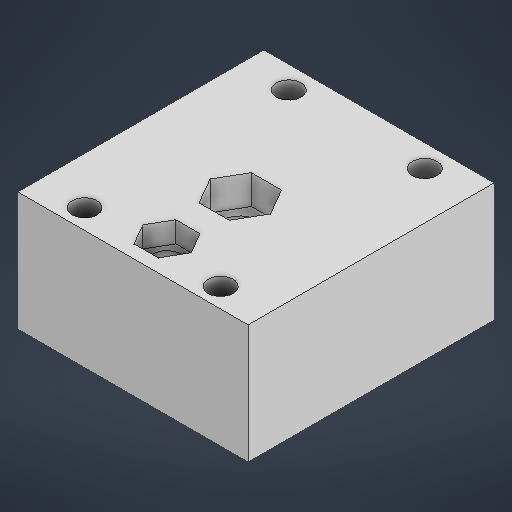
# Autodesk Inventor part: adapter-optical
Saved by Autodesk Inventor 2026.2 (Build 302298000, 298)
## iProperties
Created: 2026-05-22
Part Number: adapter-optical
Material: Generic
Document SubType Name: Modeling
Designer: mayhe
Density: 1 g/cm^3
Appearance: Default
Author: mayhe
Autodesk Inventor part; units mm, degrees
ref_plane "YZ Plane" through (0, 0, 0) normal (1, 0, 0) x (0, 1, 0)
ref_plane "XZ Plane" through (0, 0, 0) normal (0, 1, 0) x (-1, 0, 0)
ref_plane "XY Plane" through (0, 0, 0) normal (0, 0, 1) x (1, 0, 0)
sketch "Sketch1" plane through (0, 0, 0) normal (1, 0, 0) x (0, 1, 0)
  line L0 (11.35, 23.5) -> (-11.35, 23.5)
  line L1 (-11.35, 23.5) -> (-11.35, -23.5)
  line L2 (-11.35, -23.5) -> (11.35, -23.5)
  line L3 (11.35, -23.5) -> (11.35, 23.5)
  line L4 (11.35, 23.5) -> (-11.35, -23.5) construction
  line L5 (-11.35, 23.5) -> (11.35, -23.5) construction
  point P0 (0, 0)
  dimension "d0" = 22.7
  dimension "d1" = 47
  constraints: 12 end point, 2 midpoint, 2 parallel, 1 horizontal, 1 perpendicular
  measures "d0" distance of L2.end L1.end
  measures "d1" distance of L1.end L0.end
extrude "Extrusion1" add sketch "Sketch1" along normal mid plane 44
sketch "Sketch4" plane through (-22, -11.35, 23.5) normal (0, 1, 0) x (1, 0, 0)
  circle A0 centre (9, 42.75) radius 2.375
  line L0 (0, 47) -> (44, 47) projected
  line L1 (0, 0) -> (0, 47) projected
  circle A1 centre (35, 42.75) radius 2.375
  circle A2 centre (9, 3.75) radius 2.375
  circle A3 centre (35, 3.75) radius 2.375
  point P0 (22, 23.5)
  dimension "d23" = 4.75
  dimension "d24" = 4.25
  dimension "d25" = 9
  dimension "d28" = 26
  dimension "d31" = 39
  constraints: 4 centre point, 1 horizontal, 1 vertical, 6 other
  measures "d23" diameter of A0
  measures "d24" distance from line of L0 A0.centre
  measures "d25" distance from line of L1 A0.centre
  measures "d28" distance of A0.centre A1.centre
  measures "d31" distance of A0.centre A2.centre
hole "Event Camera mounting bolts" at (13, -11.35, -19.25) at (-13, -11.35, -19.25) at (-13, -11.35, 19.75) at (13, -11.35, 19.75) direction (0, 1, 0) diameter 4.75 depth 22.7 tip angle 118 counterbore diameter 6.5 counterbore depth 3
sketch "Sketch5" plane through (-22, -11.35, -23.5) normal (0, -1, 0) x (1, 0, 0)
  circle A0 centre (22, 40.5) radius 2
  circle A1 centre (22, 26.5) radius 2.5
  line L0 (44, 47) -> (0, 47) projected
  point P0 (22, 23.5)
  dimension "d41" = 4
  dimension "d42" = 5
  dimension "d43" = 14
  dimension "d44" = 6.5
  constraints: 2 centre point
  measures "d41" diameter of A0
  measures "d42" diameter of A1
  measures "d43" distance of A0.centre A1.centre
  measures "d44" distance from line of L0 A0.centre
hole "Small Hole" at (0, -11.35, 17) direction (0, 1, 0) diameter 5.75 depth 22.7 tip angle 118
hole "Big Hole" at (0, -11.35, 3) direction (0, 1, 0) diameter 6.75 depth 22.7 tip angle 118
sketch "Sketch6" plane through (-22, 11.35, 23.5) normal (0, 1, 0) x (1, 0, 0)
  circle A0 centre (22, 20.5) radius 3.375 projected
  circle A1 centre (22, 20.5) radius 5
  circle A2 centre (22, 6.5) radius 2.875 projected
  circle A3 centre (22, 6.5) radius 4
  line L0 (19.1132, 15.5) -> (16.2265, 20.5)
  line L1 (16.2265, 20.5) -> (19.1132, 25.5)
  line L2 (19.1132, 25.5) -> (24.8868, 25.5)
  line L3 (24.8868, 25.5) -> (27.7735, 20.5)
  line L4 (27.7735, 20.5) -> (24.8868, 15.5)
  line L5 (24.8868, 15.5) -> (19.1132, 15.5)
  line L6 (19.689, 2.5009) -> (17.3812, 6.5019)
  line L7 (17.3812, 6.5019) -> (19.6922, 10.5009)
  line L8 (19.6922, 10.5009) -> (24.311, 10.4991)
  line L9 (24.311, 10.4991) -> (26.6188, 6.4981)
  line L10 (26.6188, 6.4981) -> (24.3078, 2.4991)
  line L11 (24.3078, 2.4991) -> (19.689, 2.5009)
  point P0 (22, 23.5)
  point P1 (22, 15.5)
  point P2 (21.9984, 2.5)
  dimension "d59" = 10
  dimension "d60" = 8
  constraints: 24 end point, 4 coincident, 2 midpoint, 1 vertical alignment, 31 other
extrude "Big Hole Nut" cut sketch "Sketch6" against normal blind 5.6 contours A0 | A1 | A1 L3 L4 | A1 L2 L3 | L4 L5 A1 | A1 L1 L2 | L5 L0 A1 | A1 L0 L1
extrude "Small Hole Nut" cut sketch "Sketch6" against normal blind 4 contours A2 | A3 | A3 L9 L10 | A3 L8 L9 | L10 L11 A3 | A3 L7 L8 | L11 L6 A3 | A3 L6 L7
sketch "Sketch8" plane through (22, 11.35, -23.5) normal (0, 0, -1) x (-1, 0, 0)
  line L0 (-7.9257, -5.0636) -> (51.9257, -5.0636) construction
  line L1 (51.9257, -5.0636) -> (51.9257, -17.6364) construction
  line L2 (51.9257, -17.6364) -> (-7.9257, -17.6364) construction
  line L3 (-7.9257, -17.6364) -> (-7.9257, -5.0636) construction
  line L4 (24.8868, 0) -> (19.1132, 0) projected
  line L5 (22, 0) -> (22, -22.7)
  line L6 (44, -22.7) -> (0, -22.7) projected
  line L7 (44, 0) -> (0, 0) projected
  line L8 (1.4952, -10.1017) -> (1.4952, -7.0537)
  line L9 (1.4952, -7.0537) -> (3.402, -7.0537)
  line L10 (3.402, -7.0537) -> (3.402, -7.4143)
  line L11 (3.402, -7.4143) -> (1.9002, -7.4143)
  line L12 (1.9002, -7.4143) -> (1.9002, -8.2492)
  line L13 (1.9002, -8.2492) -> (3.3007, -8.2492)
  line L14 (3.3007, -8.2492) -> (3.3007, -8.6098)
  line L15 (3.3007, -8.6098) -> (1.9002, -8.6098)
  line L16 (1.9002, -8.6098) -> (1.9002, -9.7411)
  line L17 (1.9002, -9.7411) -> (3.402, -9.7411)
  line L18 (3.402, -9.7411) -> (3.402, -10.1017)
  line L19 (3.402, -10.1017) -> (1.4952, -10.1017)
  line L20 (5.6127, -7.8145) -> (4.7506, -10.1017)
  line L21 (4.7506, -10.1017) -> (4.4048, -10.1017)
  line L22 (4.4048, -10.1017) -> (3.5502, -7.8145)
  line L23 (3.5502, -7.8145) -> (3.9676, -7.8145)
  line L24 (3.9676, -7.8145) -> (4.5926, -9.5756)
  line L25 (4.5926, -9.5756) -> (5.2125, -7.8145)
  line L26 (5.2125, -7.8145) -> (5.6127, -7.8145)
  spline S0 degree 2 poles (6.8971, -10.1536) (6.3487, -10.1536) (5.7461, -9.5386) (5.7461, -8.9704) knots 0 0 0 1 2 2 2
  spline S1 degree 2 poles (5.7461, -8.9704) (5.7461, -8.4122) (6.3315, -7.7503) (6.8032, -7.7503) knots 0 0 0 1 2 2 2
  spline S2 degree 2 poles (6.8032, -7.7503) (7.0156, -7.7503) (7.3442, -7.8738) (7.4652, -8.0047) knots 0 0 0 1 2 2 2
  spline S3 degree 2 poles (7.4652, -8.0047) (7.5887, -8.1356) (7.7196, -8.5135) (7.7196, -8.7877) knots 0 0 0 1 2 2 2
  line L27 (7.7196, -8.7877) -> (7.7196, -8.9976)
  line L28 (7.7196, -8.9976) -> (6.1363, -8.9976)
  spline S4 degree 2 poles (6.1363, -8.9976) (6.1363, -9.3953) (6.5365, -9.8177) (6.8921, -9.8177) knots 0 0 0 1 2 2 2
  spline S5 degree 2 poles (6.8921, -9.8177) (7.0181, -9.8177) (7.2626, -9.7609) (7.3614, -9.7164) knots 0 0 0 1 2 2 2
  spline S6 degree 2 poles (7.3614, -9.7164) (7.4652, -9.667) (7.6085, -9.5805) (7.6554, -9.541) knots 0 0 0 1 2 2 2
  line L29 (7.6554, -9.541) -> (7.6776, -9.541)
  line L30 (7.6776, -9.541) -> (7.6776, -9.9609)
  spline S7 degree 2 poles (7.6776, -9.9609) (7.6109, -9.9881) (7.4084, -10.0671) (7.3293, -10.0894) knots 0 0 0 1 2 2 2
  spline S8 degree 2 poles (7.3293, -10.0894) (7.2182, -10.1215) (7.0354, -10.1536) (6.8971, -10.1536) knots 0 0 0 1 2 2 2
  spline S9 degree 2 poles (7.3442, -8.7037) (7.3392, -8.5481) (7.275, -8.3208) (7.2132, -8.2443) knots 0 0 0 1 2 2 2
  spline S10 degree 2 poles (7.2132, -8.2443) (7.1466, -8.1578) (6.9366, -8.0664) (6.781, -8.0664) knots 0 0 0 1 2 2 2
  spline S11 degree 2 poles (6.781, -8.0664) (6.6279, -8.0664) (6.413, -8.1578) (6.324, -8.2467) knots 0 0 0 1 2 2 2
  spline S12 degree 2 poles (6.324, -8.2467) (6.2376, -8.3381) (6.1487, -8.558) (6.1363, -8.7037) knots 0 0 0 1 2 2 2
  line L31 (6.1363, -8.7037) -> (7.3442, -8.7037)
  line L32 (9.9056, -10.1017) -> (9.5202, -10.1017)
  line L33 (9.5202, -10.1017) -> (9.5202, -8.7975)
  spline S13 degree 2 poles (9.5202, -8.7975) (9.5202, -8.6395) (9.4906, -8.3678) (9.4461, -8.2863) knots 0 0 0 1 2 2 2
  spline S14 degree 2 poles (9.4461, -8.2863) (9.3992, -8.1998) (9.2313, -8.1158) (9.088, -8.1158) knots 0 0 0 1 2 2 2
  spline S15 degree 2 poles (9.088, -8.1158) (8.9447, -8.1158) (8.6409, -8.269) (8.4952, -8.3925) knots 0 0 0 1 2 2 2
  line L34 (8.4952, -8.3925) -> (8.4952, -10.1017)
  line L35 (8.4952, -10.1017) -> (8.1099, -10.1017)
  line L36 (8.1099, -10.1017) -> (8.1099, -7.8145)
  line L37 (8.1099, -7.8145) -> (8.4952, -7.8145)
  line L38 (8.4952, -7.8145) -> (8.4952, -8.0689)
  spline S16 degree 2 poles (8.4952, -8.0689) (8.6681, -7.9133) (9.0015, -7.7503) (9.1893, -7.7503) knots 0 0 0 1 2 2 2
  spline S17 degree 2 poles (9.1893, -7.7503) (9.5252, -7.7503) (9.9056, -8.1949) (9.9056, -8.6172) knots 0 0 0 1 2 2 2
  line L39 (9.9056, -8.6172) -> (9.9056, -10.1017)
  spline S18 degree 2 poles (11.1381, -10.1462) (10.8244, -10.1462) (10.4712, -9.788) (10.4712, -9.4002) knots 0 0 0 1 2 2 2
  line L40 (10.4712, -9.4002) -> (10.4712, -8.1331)
  line L41 (10.4712, -8.1331) -> (10.2118, -8.1331)
  line L42 (10.2118, -8.1331) -> (10.2118, -7.8145)
  line L43 (10.2118, -7.8145) -> (10.4712, -7.8145)
  line L44 (10.4712, -7.8145) -> (10.4712, -7.1575)
  line L45 (10.4712, -7.1575) -> (10.8565, -7.1575)
  line L46 (10.8565, -7.1575) -> (10.8565, -7.8145)
  line L47 (10.8565, -7.8145) -> (11.5654, -7.8145)
  line L48 (11.5654, -7.8145) -> (11.5654, -8.1331)
  line L49 (11.5654, -8.1331) -> (10.8565, -8.1331)
  line L50 (10.8565, -8.1331) -> (10.8565, -9.2224)
  spline S19 degree 2 poles (10.8565, -9.2224) (10.8565, -9.3953) (10.8689, -9.5855) (10.9109, -9.667) knots 0 0 0 1 2 2 2
  spline S20 degree 2 poles (10.9109, -9.667) (10.9454, -9.7386) (11.1011, -9.8103) (11.2344, -9.8103) knots 0 0 0 1 2 2 2
  spline S21 degree 2 poles (11.2344, -9.8103) (11.3283, -9.8103) (11.5037, -9.7534) (11.5432, -9.7362) knots 0 0 0 1 2 2 2
  line L51 (11.5432, -9.7362) -> (11.5654, -9.7362)
  line L52 (11.5654, -9.7362) -> (11.5654, -10.082)
  spline S22 degree 2 poles (11.5654, -10.082) (11.4567, -10.1116) (11.2344, -10.1462) (11.1381, -10.1462) knots 0 0 0 1 2 2 2
  spline S23 degree 2 poles (14.3788, -10.1561) (14.0824, -10.1561) (13.581, -9.956) (13.3982, -9.7559) knots 0 0 0 1 2 2 2
  spline S24 degree 2 poles (13.3982, -9.7559) (13.2154, -9.5583) (13.0153, -8.9655) (13.0153, -8.5802) knots 0 0 0 1 2 2 2
  spline S25 degree 2 poles (13.0153, -8.5802) (13.0153, -8.1973) (13.2104, -7.6292) (13.3957, -7.4193) knots 0 0 0 1 2 2 2
  spline S26 degree 2 poles (13.3957, -7.4193) (13.5785, -7.2143) (14.0774, -6.9994) (14.3862, -6.9994) knots 0 0 0 1 2 2 2
  spline S27 degree 2 poles (14.3862, -6.9994) (14.5393, -6.9994) (14.8085, -7.0438) (14.9222, -7.0784) knots 0 0 0 1 2 2 2
  spline S28 degree 2 poles (14.9222, -7.0784) (15.021, -7.1105) (15.226, -7.2019) (15.3273, -7.2563) knots 0 0 0 1 2 2 2
  line L53 (15.3273, -7.2563) -> (15.3273, -7.7453)
  line L54 (15.3273, -7.7453) -> (15.2951, -7.7453)
  spline S29 degree 2 poles (15.2951, -7.7453) (15.2408, -7.6959) (15.0728, -7.5576) (14.9518, -7.4909) knots 0 0 0 1 2 2 2
  spline S30 degree 2 poles (14.9518, -7.4909) (14.8357, -7.4267) (14.5615, -7.3452) (14.3837, -7.3452) knots 0 0 0 1 2 2 2
  spline S31 degree 2 poles (14.3837, -7.3452) (14.1886, -7.3452) (13.8403, -7.5057) (13.7094, -7.6589) knots 0 0 0 1 2 2 2
  spline S32 degree 2 poles (13.7094, -7.6589) (13.581, -7.8145) (13.4377, -8.2863) (13.4377, -8.5802) knots 0 0 0 1 2 2 2
  spline S33 degree 2 poles (13.4377, -8.5802) (13.4377, -8.8939) (13.5884, -9.3459) (13.7193, -9.5015) knots 0 0 0 1 2 2 2
  spline S34 degree 2 poles (13.7193, -9.5015) (13.8477, -9.6522) (14.191, -9.8053) (14.3837, -9.8053) knots 0 0 0 1 2 2 2
  spline S35 degree 2 poles (14.3837, -9.8053) (14.5591, -9.8053) (14.8579, -9.7189) (14.974, -9.6546) knots 0 0 0 1 2 2 2
  spline S36 degree 2 poles (14.974, -9.6546) (15.0852, -9.5904) (15.2507, -9.457) (15.2976, -9.4101) knots 0 0 0 1 2 2 2
  line L55 (15.2976, -9.4101) -> (15.3273, -9.4101)
  line L56 (15.3273, -9.4101) -> (15.3273, -9.8942)
  spline S37 degree 2 poles (15.3273, -9.8942) (15.226, -9.9412) (15.0481, -10.0276) (14.9222, -10.0671) knots 0 0 0 1 2 2 2
  spline S38 degree 2 poles (14.9222, -10.0671) (14.7888, -10.1116) (14.5615, -10.1561) (14.3788, -10.1561) knots 0 0 0 1 2 2 2
  spline S39 degree 2 poles (16.9501, -9.8597) (16.9031, -9.8942) (16.745, -10.0177) (16.6709, -10.0548) knots 0 0 0 1 2 2 2
  spline S40 degree 2 poles (16.6709, -10.0548) (16.5697, -10.1091) (16.3795, -10.1659) (16.2066, -10.1659) knots 0 0 0 1 2 2 2
  spline S41 degree 2 poles (16.2066, -10.1659) (16.0658, -10.1659) (15.8114, -10.0597) (15.715, -9.9634) knots 0 0 0 1 2 2 2
  spline S42 degree 2 poles (15.715, -9.9634) (15.6237, -9.8695) (15.5125, -9.5929) (15.5125, -9.4398) knots 0 0 0 1 2 2 2
  spline S43 degree 2 poles (15.5125, -9.4398) (15.5125, -9.2026) (15.7126, -8.8667) (15.9299, -8.7704) knots 0 0 0 1 2 2 2
  spline S44 degree 2 poles (15.9299, -8.7704) (16.1226, -8.6815) (16.6462, -8.6148) (16.9501, -8.5975) knots 0 0 0 1 2 2 2
  line L57 (16.9501, -8.5975) -> (16.9501, -8.5234)
  spline S45 degree 2 poles (16.9501, -8.5234) (16.9501, -8.39) (16.8685, -8.2245) (16.7944, -8.1776) knots 0 0 0 1 2 2 2
  spline S46 degree 2 poles (16.7944, -8.1776) (16.7203, -8.1306) (16.5079, -8.101) (16.3943, -8.101) knots 0 0 0 1 2 2 2
  spline S47 degree 2 poles (16.3943, -8.101) (16.2609, -8.101) (15.9003, -8.18) (15.72, -8.2566) knots 0 0 0 1 2 2 2
  line L58 (15.72, -8.2566) -> (15.6978, -8.2566)
  line L59 (15.6978, -8.2566) -> (15.6978, -7.8639)
  spline S48 degree 2 poles (15.6978, -7.8639) (15.804, -7.8342) (16.2016, -7.7601) (16.3968, -7.7601) knots 0 0 0 1 2 2 2
  spline S49 degree 2 poles (16.3968, -7.7601) (16.6339, -7.7601) (16.9575, -7.8342) (17.0859, -7.9306) knots 0 0 0 1 2 2 2
  spline S50 degree 2 poles (17.0859, -7.9306) (17.2119, -8.0244) (17.3354, -8.3233) (17.3354, -8.5382) knots 0 0 0 1 2 2 2
  line L60 (17.3354, -8.5382) -> (17.3354, -10.1017)
  line L61 (17.3354, -10.1017) -> (16.9501, -10.1017)
  line L62 (16.9501, -10.1017) -> (16.9501, -9.8597)
  line L63 (16.9501, -9.5386) -> (16.9501, -8.9038)
  spline S51 degree 2 poles (16.9501, -8.9038) (16.8117, -8.9161) (16.3943, -8.9581) (16.2634, -8.9976) knots 0 0 0 1 2 2 2
  spline S52 degree 2 poles (16.2634, -8.9976) (16.1102, -9.0446) (15.9102, -9.2397) (15.9102, -9.4126) knots 0 0 0 1 2 2 2
  spline S53 degree 2 poles (15.9102, -9.4126) (15.9102, -9.6102) (16.1325, -9.8103) (16.3449, -9.8103) knots 0 0 0 1 2 2 2
  spline S54 degree 2 poles (16.3449, -9.8103) (16.5252, -9.8103) (16.8216, -9.6546) (16.9501, -9.5386) knots 0 0 0 1 2 2 2
  line L64 (20.4698, -10.1017) -> (20.4698, -8.7778)
  spline S55 degree 2 poles (20.4698, -8.7778) (20.4698, -8.6197) (20.4451, -8.3505) (20.4056, -8.2764) knots 0 0 0 1 2 2 2
  spline S56 degree 2 poles (20.4056, -8.2764) (20.3661, -8.1949) (20.2154, -8.1158) (20.0845, -8.1158) knots 0 0 0 1 2 2 2
  spline S57 degree 2 poles (20.0845, -8.1158) (19.9659, -8.1158) (19.6942, -8.2616) (19.551, -8.3999) knots 0 0 0 1 2 2 2
  spline S58 degree 2 poles (19.551, -8.3999) (19.5534, -8.4345) (19.5584, -8.5308) (19.5584, -8.595) knots 0 0 0 1 2 2 2
  line L65 (19.5584, -8.595) -> (19.5584, -10.1017)
  line L66 (19.5584, -10.1017) -> (19.1731, -10.1017)
  line L67 (19.1731, -10.1017) -> (19.1731, -8.7778)
  spline S59 degree 2 poles (19.1731, -8.7778) (19.1731, -8.6197) (19.1484, -8.3505) (19.1088, -8.2764) knots 0 0 0 1 2 2 2
  spline S60 degree 2 poles (19.1088, -8.2764) (19.0693, -8.1949) (18.9187, -8.1158) (18.7877, -8.1158) knots 0 0 0 1 2 2 2
  spline S61 degree 2 poles (18.7877, -8.1158) (18.6642, -8.1158) (18.3901, -8.2714) (18.2616, -8.3925) knots 0 0 0 1 2 2 2
  line L68 (18.2616, -8.3925) -> (18.2616, -10.1017)
  line L69 (18.2616, -10.1017) -> (17.8763, -10.1017)
  line L70 (17.8763, -10.1017) -> (17.8763, -7.8145)
  line L71 (17.8763, -7.8145) -> (18.2616, -7.8145)
  line L72 (18.2616, -7.8145) -> (18.2616, -8.0664)
  spline S62 degree 2 poles (18.2616, -8.0664) (18.4123, -7.9158) (18.7087, -7.7503) (18.8865, -7.7503) knots 0 0 0 1 2 2 2
  spline S63 degree 2 poles (18.8865, -7.7503) (19.0891, -7.7503) (19.4028, -7.9355) (19.4843, -8.1455) knots 0 0 0 1 2 2 2
  spline S64 degree 2 poles (19.4843, -8.1455) (19.6597, -7.9503) (19.9906, -7.7503) (20.1833, -7.7503) knots 0 0 0 1 2 2 2
  spline S65 degree 2 poles (20.1833, -7.7503) (20.3315, -7.7503) (20.5736, -7.8417) (20.6625, -7.9454) knots 0 0 0 1 2 2 2
  spline S66 degree 2 poles (20.6625, -7.9454) (20.7539, -8.0491) (20.8551, -8.3604) (20.8551, -8.595) knots 0 0 0 1 2 2 2
  line L73 (20.8551, -8.595) -> (20.8551, -10.1017)
  line L74 (20.8551, -10.1017) -> (20.4698, -10.1017)
  spline S67 degree 2 poles (22.389, -10.1536) (21.8407, -10.1536) (21.238, -9.5386) (21.238, -8.9704) knots 0 0 0 1 2 2 2
  spline S68 degree 2 poles (21.238, -8.9704) (21.238, -8.4122) (21.8234, -7.7503) (22.2952, -7.7503) knots 0 0 0 1 2 2 2
  spline S69 degree 2 poles (22.2952, -7.7503) (22.5076, -7.7503) (22.8361, -7.8738) (22.9571, -8.0047) knots 0 0 0 1 2 2 2
  spline S70 degree 2 poles (22.9571, -8.0047) (23.0806, -8.1356) (23.2115, -8.5135) (23.2115, -8.7877) knots 0 0 0 1 2 2 2
  line L75 (23.2115, -8.7877) -> (23.2115, -8.9976)
  line L76 (23.2115, -8.9976) -> (21.6283, -8.9976)
  spline S71 degree 2 poles (21.6283, -8.9976) (21.6283, -9.3953) (22.0284, -9.8177) (22.3841, -9.8177) knots 0 0 0 1 2 2 2
  spline S72 degree 2 poles (22.3841, -9.8177) (22.5101, -9.8177) (22.7546, -9.7609) (22.8534, -9.7164) knots 0 0 0 1 2 2 2
  spline S73 degree 2 poles (22.8534, -9.7164) (22.9571, -9.667) (23.1004, -9.5805) (23.1473, -9.541) knots 0 0 0 1 2 2 2
  line L77 (23.1473, -9.541) -> (23.1696, -9.541)
  line L78 (23.1696, -9.541) -> (23.1696, -9.9609)
  spline S74 degree 2 poles (23.1696, -9.9609) (23.1029, -9.9881) (22.9003, -10.0671) (22.8213, -10.0894) knots 0 0 0 1 2 2 2
  spline S75 degree 2 poles (22.8213, -10.0894) (22.7101, -10.1215) (22.5273, -10.1536) (22.389, -10.1536) knots 0 0 0 1 2 2 2
  spline S76 degree 2 poles (22.8361, -8.7037) (22.8312, -8.5481) (22.7669, -8.3208) (22.7052, -8.2443) knots 0 0 0 1 2 2 2
  spline S77 degree 2 poles (22.7052, -8.2443) (22.6385, -8.1578) (22.4285, -8.0664) (22.2729, -8.0664) knots 0 0 0 1 2 2 2
  spline S78 degree 2 poles (22.2729, -8.0664) (22.1198, -8.0664) (21.9049, -8.1578) (21.816, -8.2467) knots 0 0 0 1 2 2 2
  spline S79 degree 2 poles (21.816, -8.2467) (21.7295, -8.3381) (21.6406, -8.558) (21.6283, -8.7037) knots 0 0 0 1 2 2 2
  line L79 (21.6283, -8.7037) -> (22.8361, -8.7037)
  line L80 (24.8146, -8.227) -> (24.7948, -8.227)
  spline S80 degree 2 poles (24.7948, -8.227) (24.7504, -8.2146) (24.654, -8.2097) (24.5873, -8.2097) knots 0 0 0 1 2 2 2
  spline S81 degree 2 poles (24.5873, -8.2097) (24.4317, -8.2097) (24.1254, -8.3455) (23.9871, -8.4789) knots 0 0 0 1 2 2 2
  line L81 (23.9871, -8.4789) -> (23.9871, -10.1017)
  line L82 (23.9871, -10.1017) -> (23.6018, -10.1017)
  line L83 (23.6018, -10.1017) -> (23.6018, -7.8145)
  line L84 (23.6018, -7.8145) -> (23.9871, -7.8145)
  line L85 (23.9871, -7.8145) -> (23.9871, -8.1553)
  spline S82 degree 2 poles (23.9871, -8.1553) (24.1971, -7.9676) (24.5108, -7.8145) (24.659, -7.8145) knots 0 0 0 1 2 2 2
  spline S83 degree 2 poles (24.659, -7.8145) (24.7183, -7.8145) (24.7775, -7.8194) (24.8146, -7.8268) knots 0 0 0 1 2 2 2
  line L86 (24.8146, -7.8268) -> (24.8146, -8.227)
  spline S84 degree 2 poles (26.388, -9.8597) (26.3411, -9.8942) (26.183, -10.0177) (26.1089, -10.0548) knots 0 0 0 1 2 2 2
  spline S85 degree 2 poles (26.1089, -10.0548) (26.0076, -10.1091) (25.8174, -10.1659) (25.6445, -10.1659) knots 0 0 0 1 2 2 2
  spline S86 degree 2 poles (25.6445, -10.1659) (25.5037, -10.1659) (25.2493, -10.0597) (25.153, -9.9634) knots 0 0 0 1 2 2 2
  spline S87 degree 2 poles (25.153, -9.9634) (25.0616, -9.8695) (24.9504, -9.5929) (24.9504, -9.4398) knots 0 0 0 1 2 2 2
  spline S88 degree 2 poles (24.9504, -9.4398) (24.9504, -9.2026) (25.1505, -8.8667) (25.3679, -8.7704) knots 0 0 0 1 2 2 2
  spline S89 degree 2 poles (25.3679, -8.7704) (25.5605, -8.6815) (26.0842, -8.6148) (26.388, -8.5975) knots 0 0 0 1 2 2 2
  line L87 (26.388, -8.5975) -> (26.388, -8.5234)
  spline S90 degree 2 poles (26.388, -8.5234) (26.388, -8.39) (26.3065, -8.2245) (26.2324, -8.1776) knots 0 0 0 1 2 2 2
  spline S91 degree 2 poles (26.2324, -8.1776) (26.1583, -8.1306) (25.9459, -8.101) (25.8322, -8.101) knots 0 0 0 1 2 2 2
  spline S92 degree 2 poles (25.8322, -8.101) (25.6988, -8.101) (25.3382, -8.18) (25.1579, -8.2566) knots 0 0 0 1 2 2 2
  line L88 (25.1579, -8.2566) -> (25.1357, -8.2566)
  line L89 (25.1357, -8.2566) -> (25.1357, -7.8639)
  spline S93 degree 2 poles (25.1357, -7.8639) (25.2419, -7.8342) (25.6396, -7.7601) (25.8347, -7.7601) knots 0 0 0 1 2 2 2
  spline S94 degree 2 poles (25.8347, -7.7601) (26.0718, -7.7601) (26.3954, -7.8342) (26.5238, -7.9306) knots 0 0 0 1 2 2 2
  spline S95 degree 2 poles (26.5238, -7.9306) (26.6498, -8.0244) (26.7733, -8.3233) (26.7733, -8.5382) knots 0 0 0 1 2 2 2
  line L90 (26.7733, -8.5382) -> (26.7733, -10.1017)
  line L91 (26.7733, -10.1017) -> (26.388, -10.1017)
  line L92 (26.388, -10.1017) -> (26.388, -9.8597)
  line L93 (26.388, -9.5386) -> (26.388, -8.9038)
  spline S96 degree 2 poles (26.388, -8.9038) (26.2497, -8.9161) (25.8322, -8.9581) (25.7013, -8.9976) knots 0 0 0 1 2 2 2
  spline S97 degree 2 poles (25.7013, -8.9976) (25.5482, -9.0446) (25.3481, -9.2397) (25.3481, -9.4126) knots 0 0 0 1 2 2 2
  spline S98 degree 2 poles (25.3481, -9.4126) (25.3481, -9.6102) (25.5704, -9.8103) (25.7828, -9.8103) knots 0 0 0 1 2 2 2
  spline S99 degree 2 poles (25.7828, -9.8103) (25.9631, -9.8103) (26.2595, -9.6546) (26.388, -9.5386) knots 0 0 0 1 2 2 2
  line L94 (28.3245, -10.1017) -> (29.352, -7.0537)
  line L95 (29.352, -7.0537) -> (29.8509, -7.0537)
  line L96 (29.8509, -7.0537) -> (30.8785, -10.1017)
  line L97 (30.8785, -10.1017) -> (30.4512, -10.1017)
  line L98 (30.4512, -10.1017) -> (30.1745, -9.2496)
  line L99 (30.1745, -9.2496) -> (29.0111, -9.2496)
  line L100 (29.0111, -9.2496) -> (28.7345, -10.1017)
  line L101 (28.7345, -10.1017) -> (28.3245, -10.1017)
  line L102 (30.0634, -8.9038) -> (29.5916, -7.4687)
  line L103 (29.5916, -7.4687) -> (29.1223, -8.9038)
  line L104 (29.1223, -8.9038) -> (30.0634, -8.9038)
  line L105 (32.8965, -10.1017) -> (32.5112, -10.1017)
  line L106 (32.5112, -10.1017) -> (32.5112, -9.8695)
  spline S100 degree 2 poles (32.5112, -9.8695) (32.4222, -9.9436) (32.2913, -10.0424) (32.2024, -10.0844) knots 0 0 0 1 2 2 2
  spline S101 degree 2 poles (32.2024, -10.0844) (32.1209, -10.1239) (31.9455, -10.1659) (31.8294, -10.1659) knots 0 0 0 1 2 2 2
  spline S102 degree 2 poles (31.8294, -10.1659) (31.6417, -10.1659) (31.3255, -10.0103) (31.2144, -9.8597) knots 0 0 0 1 2 2 2
  spline S103 degree 2 poles (31.2144, -9.8597) (31.1032, -9.709) (30.9797, -9.2644) (30.9797, -8.9754) knots 0 0 0 1 2 2 2
  spline S104 degree 2 poles (30.9797, -8.9754) (30.9797, -8.674) (31.1354, -8.2344) (31.2712, -8.0689) knots 0 0 0 1 2 2 2
  spline S105 degree 2 poles (31.2712, -8.0689) (31.3972, -7.9207) (31.7504, -7.7503) (31.9455, -7.7503) knots 0 0 0 1 2 2 2
  spline S106 degree 2 poles (31.9455, -7.7503) (32.116, -7.7503) (32.3704, -7.8268) (32.5112, -7.9059) knots 0 0 0 1 2 2 2
  line L107 (32.5112, -7.9059) -> (32.5112, -6.9179)
  line L108 (32.5112, -6.9179) -> (32.8965, -6.9179)
  line L109 (32.8965, -6.9179) -> (32.8965, -10.1017)
  line L110 (32.5112, -9.546) -> (32.5112, -8.2245)
  spline S107 degree 2 poles (32.5112, -8.2245) (32.3679, -8.1553) (32.1407, -8.1035) (32.0097, -8.1035) knots 0 0 0 1 2 2 2
  spline S108 degree 2 poles (32.0097, -8.1035) (31.7133, -8.1035) (31.3774, -8.5481) (31.3774, -8.968) knots 0 0 0 1 2 2 2
  spline S109 degree 2 poles (31.3774, -8.968) (31.3774, -9.3731) (31.6343, -9.8004) (31.9184, -9.8004) knots 0 0 0 1 2 2 2
  spline S110 degree 2 poles (31.9184, -9.8004) (32.069, -9.8004) (32.3753, -9.6621) (32.5112, -9.546) knots 0 0 0 1 2 2 2
  spline S111 degree 2 poles (34.7292, -9.8597) (34.6823, -9.8942) (34.5242, -10.0177) (34.4501, -10.0548) knots 0 0 0 1 2 2 2
  spline S112 degree 2 poles (34.4501, -10.0548) (34.3488, -10.1091) (34.1587, -10.1659) (33.9858, -10.1659) knots 0 0 0 1 2 2 2
  spline S113 degree 2 poles (33.9858, -10.1659) (33.845, -10.1659) (33.5906, -10.0597) (33.4942, -9.9634) knots 0 0 0 1 2 2 2
  spline S114 degree 2 poles (33.4942, -9.9634) (33.4028, -9.8695) (33.2917, -9.5929) (33.2917, -9.4398) knots 0 0 0 1 2 2 2
  spline S115 degree 2 poles (33.2917, -9.4398) (33.2917, -9.2026) (33.4918, -8.8667) (33.7091, -8.7704) knots 0 0 0 1 2 2 2
  spline S116 degree 2 poles (33.7091, -8.7704) (33.9018, -8.6815) (34.4254, -8.6148) (34.7292, -8.5975) knots 0 0 0 1 2 2 2
  line L111 (34.7292, -8.5975) -> (34.7292, -8.5234)
  spline S117 degree 2 poles (34.7292, -8.5234) (34.7292, -8.39) (34.6477, -8.2245) (34.5736, -8.1776) knots 0 0 0 1 2 2 2
  spline S118 degree 2 poles (34.5736, -8.1776) (34.4995, -8.1306) (34.2871, -8.101) (34.1735, -8.101) knots 0 0 0 1 2 2 2
  spline S119 degree 2 poles (34.1735, -8.101) (34.0401, -8.101) (33.6795, -8.18) (33.4992, -8.2566) knots 0 0 0 1 2 2 2
  line L112 (33.4992, -8.2566) -> (33.4769, -8.2566)
  line L113 (33.4769, -8.2566) -> (33.4769, -7.8639)
  spline S120 degree 2 poles (33.4769, -7.8639) (33.5831, -7.8342) (33.9808, -7.7601) (34.1759, -7.7601) knots 0 0 0 1 2 2 2
  spline S121 degree 2 poles (34.1759, -7.7601) (34.4131, -7.7601) (34.7366, -7.8342) (34.8651, -7.9306) knots 0 0 0 1 2 2 2
  spline S122 degree 2 poles (34.8651, -7.9306) (34.9911, -8.0244) (35.1146, -8.3233) (35.1146, -8.5382) knots 0 0 0 1 2 2 2
  line L114 (35.1146, -8.5382) -> (35.1146, -10.1017)
  line L115 (35.1146, -10.1017) -> (34.7292, -10.1017)
  line L116 (34.7292, -10.1017) -> (34.7292, -9.8597)
  line L117 (34.7292, -9.5386) -> (34.7292, -8.9038)
  spline S123 degree 2 poles (34.7292, -8.9038) (34.5909, -8.9161) (34.1735, -8.9581) (34.0426, -8.9976) knots 0 0 0 1 2 2 2
  spline S124 degree 2 poles (34.0426, -8.9976) (33.8894, -9.0446) (33.6894, -9.2397) (33.6894, -9.4126) knots 0 0 0 1 2 2 2
  spline S125 degree 2 poles (33.6894, -9.4126) (33.6894, -9.6102) (33.9117, -9.8103) (34.1241, -9.8103) knots 0 0 0 1 2 2 2
  spline S126 degree 2 poles (34.1241, -9.8103) (34.3044, -9.8103) (34.6008, -9.6546) (34.7292, -9.5386) knots 0 0 0 1 2 2 2
  spline S127 degree 2 poles (37.5722, -8.8963) (37.5722, -9.4694) (37.0263, -10.1462) (36.6089, -10.1462) knots 0 0 0 1 2 2 2
  spline S128 degree 2 poles (36.6089, -10.1462) (36.4385, -10.1462) (36.1767, -10.0671) (36.0408, -9.9856) knots 0 0 0 1 2 2 2
  line L118 (36.0408, -9.9856) -> (36.0408, -10.944)
  line L119 (36.0408, -10.944) -> (35.6555, -10.944)
  line L120 (35.6555, -10.944) -> (35.6555, -7.8145)
  line L121 (35.6555, -7.8145) -> (36.0408, -7.8145)
  line L122 (36.0408, -7.8145) -> (36.0408, -8.0541)
  spline S129 degree 2 poles (36.0408, -8.0541) (36.1841, -7.9232) (36.5348, -7.7503) (36.7398, -7.7503) knots 0 0 0 1 2 2 2
  spline S130 degree 2 poles (36.7398, -7.7503) (37.1326, -7.7503) (37.5722, -8.3727) (37.5722, -8.8963) knots 0 0 0 1 2 2 2
  spline S131 degree 2 poles (37.1745, -8.9408) (37.1745, -8.5481) (36.9251, -8.1158) (36.646, -8.1158) knots 0 0 0 1 2 2 2
  spline S132 degree 2 poles (36.646, -8.1158) (36.4829, -8.1158) (36.1767, -8.2616) (36.0408, -8.3752) knots 0 0 0 1 2 2 2
  line L123 (36.0408, -8.3752) -> (36.0408, -9.6744)
  spline S133 degree 2 poles (36.0408, -9.6744) (36.1915, -9.746) (36.4064, -9.8004) (36.5447, -9.8004) knots 0 0 0 1 2 2 2
  spline S134 degree 2 poles (36.5447, -9.8004) (36.8436, -9.8004) (37.1745, -9.3607) (37.1745, -8.9408) knots 0 0 0 1 2 2 2
  spline S135 degree 2 poles (38.664, -10.1462) (38.3503, -10.1462) (37.9971, -9.788) (37.9971, -9.4002) knots 0 0 0 1 2 2 2
  line L124 (37.9971, -9.4002) -> (37.9971, -8.1331)
  line L125 (37.9971, -8.1331) -> (37.7377, -8.1331)
  line L126 (37.7377, -8.1331) -> (37.7377, -7.8145)
  line L127 (37.7377, -7.8145) -> (37.9971, -7.8145)
  line L128 (37.9971, -7.8145) -> (37.9971, -7.1575)
  line L129 (37.9971, -7.1575) -> (38.3824, -7.1575)
  line L130 (38.3824, -7.1575) -> (38.3824, -7.8145)
  line L131 (38.3824, -7.8145) -> (39.0913, -7.8145)
  line L132 (39.0913, -7.8145) -> (39.0913, -8.1331)
  line L133 (39.0913, -8.1331) -> (38.3824, -8.1331)
  line L134 (38.3824, -8.1331) -> (38.3824, -9.2224)
  spline S136 degree 2 poles (38.3824, -9.2224) (38.3824, -9.3953) (38.3947, -9.5855) (38.4367, -9.667) knots 0 0 0 1 2 2 2
  spline S137 degree 2 poles (38.4367, -9.667) (38.4713, -9.7386) (38.6269, -9.8103) (38.7603, -9.8103) knots 0 0 0 1 2 2 2
  spline S138 degree 2 poles (38.7603, -9.8103) (38.8542, -9.8103) (39.0295, -9.7534) (39.069, -9.7362) knots 0 0 0 1 2 2 2
  line L135 (39.069, -9.7362) -> (39.0913, -9.7362)
  line L136 (39.0913, -9.7362) -> (39.0913, -10.082)
  spline S139 degree 2 poles (39.0913, -10.082) (38.9826, -10.1116) (38.7603, -10.1462) (38.664, -10.1462) knots 0 0 0 1 2 2 2
  spline S140 degree 2 poles (40.3683, -10.1536) (39.8199, -10.1536) (39.2172, -9.5386) (39.2172, -8.9704) knots 0 0 0 1 2 2 2
  spline S141 degree 2 poles (39.2172, -8.9704) (39.2172, -8.4122) (39.8026, -7.7503) (40.2744, -7.7503) knots 0 0 0 1 2 2 2
  spline S142 degree 2 poles (40.2744, -7.7503) (40.4868, -7.7503) (40.8153, -7.8738) (40.9364, -8.0047) knots 0 0 0 1 2 2 2
  spline S143 degree 2 poles (40.9364, -8.0047) (41.0599, -8.1356) (41.1908, -8.5135) (41.1908, -8.7877) knots 0 0 0 1 2 2 2
  line L137 (41.1908, -8.7877) -> (41.1908, -8.9976)
  line L138 (41.1908, -8.9976) -> (39.6075, -8.9976)
  spline S144 degree 2 poles (39.6075, -8.9976) (39.6075, -9.3953) (40.0077, -9.8177) (40.3633, -9.8177) knots 0 0 0 1 2 2 2
  spline S145 degree 2 poles (40.3633, -9.8177) (40.4893, -9.8177) (40.7338, -9.7609) (40.8326, -9.7164) knots 0 0 0 1 2 2 2
  spline S146 degree 2 poles (40.8326, -9.7164) (40.9364, -9.667) (41.0796, -9.5805) (41.1266, -9.541) knots 0 0 0 1 2 2 2
  line L139 (41.1266, -9.541) -> (41.1488, -9.541)
  line L140 (41.1488, -9.541) -> (41.1488, -9.9609)
  spline S147 degree 2 poles (41.1488, -9.9609) (41.0821, -9.9881) (40.8796, -10.0671) (40.8005, -10.0894) knots 0 0 0 1 2 2 2
  spline S148 degree 2 poles (40.8005, -10.0894) (40.6894, -10.1215) (40.5066, -10.1536) (40.3683, -10.1536) knots 0 0 0 1 2 2 2
  spline S149 degree 2 poles (40.8153, -8.7037) (40.8104, -8.5481) (40.7462, -8.3208) (40.6844, -8.2443) knots 0 0 0 1 2 2 2
  spline S150 degree 2 poles (40.6844, -8.2443) (40.6177, -8.1578) (40.4078, -8.0664) (40.2522, -8.0664) knots 0 0 0 1 2 2 2
  spline S151 degree 2 poles (40.2522, -8.0664) (40.099, -8.0664) (39.8842, -8.1578) (39.7952, -8.2467) knots 0 0 0 1 2 2 2
  spline S152 degree 2 poles (39.7952, -8.2467) (39.7088, -8.3381) (39.6199, -8.558) (39.6075, -8.7037) knots 0 0 0 1 2 2 2
  line L141 (39.6075, -8.7037) -> (40.8153, -8.7037)
  line L142 (42.7938, -8.227) -> (42.7741, -8.227)
  spline S153 degree 2 poles (42.7741, -8.227) (42.7296, -8.2146) (42.6333, -8.2097) (42.5666, -8.2097) knots 0 0 0 1 2 2 2
  spline S154 degree 2 poles (42.5666, -8.2097) (42.411, -8.2097) (42.1047, -8.3455) (41.9664, -8.4789) knots 0 0 0 1 2 2 2
  line L143 (41.9664, -8.4789) -> (41.9664, -10.1017)
  line L144 (41.9664, -10.1017) -> (41.5811, -10.1017)
  line L145 (41.5811, -10.1017) -> (41.5811, -7.8145)
  line L146 (41.5811, -7.8145) -> (41.9664, -7.8145)
  line L147 (41.9664, -7.8145) -> (41.9664, -8.1553)
  spline S155 degree 2 poles (41.9664, -8.1553) (42.1763, -7.9676) (42.49, -7.8145) (42.6382, -7.8145) knots 0 0 0 1 2 2 2
  spline S156 degree 2 poles (42.6382, -7.8145) (42.6975, -7.8145) (42.7568, -7.8194) (42.7938, -7.8268) knots 0 0 0 1 2 2 2
  line L148 (42.7938, -7.8268) -> (42.7938, -8.227)
  spline S157 degree 2 poles (14.4615, -14.1519) (14.4615, -14.3718) (14.3207, -14.7472) (14.1923, -14.8855) knots 0 0 0 1 2 2 2
  spline S158 degree 2 poles (14.1923, -14.8855) (14.0638, -15.0238) (13.681, -15.1844) (13.4439, -15.1844) knots 0 0 0 1 2 2 2
  spline S159 degree 2 poles (13.4439, -15.1844) (13.2265, -15.1844) (12.8017, -15.0881) (12.646, -15.0115) knots 0 0 0 1 2 2 2
  line L149 (12.646, -15.0115) -> (12.646, -14.5792)
  line L150 (12.646, -14.5792) -> (12.6757, -14.5792)
  spline S160 degree 2 poles (12.6757, -14.5792) (12.7226, -14.6138) (12.898, -14.7027) (13.0042, -14.7423) knots 0 0 0 1 2 2 2
  spline S161 degree 2 poles (13.0042, -14.7423) (13.1252, -14.7842) (13.3253, -14.8312) (13.4513, -14.8312) knots 0 0 0 1 2 2 2
  spline S162 degree 2 poles (13.4513, -14.8312) (13.5748, -14.8312) (13.807, -14.7423) (13.8909, -14.6459) knots 0 0 0 1 2 2 2
  spline S163 degree 2 poles (13.8909, -14.6459) (13.9675, -14.5545) (14.0465, -14.3125) (14.0465, -14.1495) knots 0 0 0 1 2 2 2
  spline S164 degree 2 poles (14.0465, -14.1495) (14.0465, -13.9864) (13.9576, -13.779) (13.8736, -13.7098) knots 0 0 0 1 2 2 2
  spline S165 degree 2 poles (13.8736, -13.7098) (13.7872, -13.6332) (13.5303, -13.569) (13.3747, -13.569) knots 0 0 0 1 2 2 2
  spline S166 degree 2 poles (13.3747, -13.569) (13.2067, -13.569) (12.8733, -13.6209) (12.772, -13.6431) knots 0 0 0 1 2 2 2
  line L151 (12.772, -13.6431) -> (12.772, -12.0722)
  line L152 (12.772, -12.0722) -> (14.4442, -12.0722)
  line L153 (14.4442, -12.0722) -> (14.4442, -12.4303)
  line L154 (14.4442, -12.4303) -> (13.1648, -12.4303)
  line L155 (13.1648, -12.4303) -> (13.1648, -13.243)
  spline S167 degree 2 poles (13.1648, -13.243) (13.2389, -13.2331) (13.3821, -13.2257) (13.4414, -13.2257) knots 0 0 0 1 2 2 2
  spline S168 degree 2 poles (13.4414, -13.2257) (13.676, -13.2257) (13.9996, -13.3022) (14.1478, -13.4159) knots 0 0 0 1 2 2 2
  spline S169 degree 2 poles (14.1478, -13.4159) (14.2985, -13.5295) (14.4615, -13.8753) (14.4615, -14.1519) knots 0 0 0 1 2 2 2
  line L156 (16.1683, -11.9363) -> (14.9753, -15.7821)
  line L157 (14.9753, -15.7821) -> (14.6295, -15.7821)
  line L158 (14.6295, -15.7821) -> (15.8175, -11.9363)
  line L159 (15.8175, -11.9363) -> (16.1683, -11.9363)
  line L160 (18.3839, -15.1202) -> (16.5042, -15.1202)
  line L161 (16.5042, -15.1202) -> (16.5042, -14.6879)
  spline S170 degree 2 poles (16.5042, -14.6879) (16.7068, -14.4977) (17.0674, -14.1445) (17.2403, -13.9543) knots 0 0 0 1 2 2 2
  spline S171 degree 2 poles (17.2403, -13.9543) (17.5886, -13.5715) (17.843, -13.112) (17.843, -12.8675) knots 0 0 0 1 2 2 2
  spline S172 degree 2 poles (17.843, -12.8675) (17.843, -12.7391) (17.7639, -12.5464) (17.6923, -12.4847) knots 0 0 0 1 2 2 2
  spline S173 degree 2 poles (17.6923, -12.4847) (17.6207, -12.4229) (17.4329, -12.3612) (17.3193, -12.3612) knots 0 0 0 1 2 2 2
  spline S174 degree 2 poles (17.3193, -12.3612) (17.2106, -12.3612) (16.9883, -12.4155) (16.8871, -12.4575) knots 0 0 0 1 2 2 2
  spline S175 degree 2 poles (16.8871, -12.4575) (16.8006, -12.4921) (16.6401, -12.5909) (16.5907, -12.6255) knots 0 0 0 1 2 2 2
  line L162 (16.5907, -12.6255) -> (16.5684, -12.6255)
  line L163 (16.5684, -12.6255) -> (16.5684, -12.1907)
  spline S176 degree 2 poles (16.5684, -12.1907) (16.6944, -12.129) (17.1464, -12.0079) (17.349, -12.0079) knots 0 0 0 1 2 2 2
  spline S177 degree 2 poles (17.349, -12.0079) (17.7763, -12.0079) (18.2579, -12.46) (18.2579, -12.8453) knots 0 0 0 1 2 2 2
  spline S178 degree 2 poles (18.2579, -12.8453) (18.2579, -13.0256) (18.1739, -13.3269) (18.0998, -13.4554) knots 0 0 0 1 2 2 2
  spline S179 degree 2 poles (18.0998, -13.4554) (18.0257, -13.5888) (17.8109, -13.8506) (17.6923, -13.9766) knots 0 0 0 1 2 2 2
  spline S180 degree 2 poles (17.6923, -13.9766) (17.4996, -14.1865) (17.0279, -14.636) (16.8871, -14.767) knots 0 0 0 1 2 2 2
  line L164 (16.8871, -14.767) -> (18.3839, -14.767)
  line L165 (18.3839, -14.767) -> (18.3839, -15.1202)
  line L166 (20.7057, -12.5291) -> (19.3867, -15.1202)
  line L167 (19.3867, -15.1202) -> (18.952, -15.1202)
  line L168 (18.952, -15.1202) -> (20.3451, -12.4303)
  line L169 (20.3451, -12.4303) -> (18.7717, -12.4303)
  line L170 (18.7717, -12.4303) -> (18.7717, -12.0722)
  line L171 (18.7717, -12.0722) -> (20.7057, -12.0722)
  line L172 (20.7057, -12.0722) -> (20.7057, -12.5291)
  line L173 (22.3458, -11.9363) -> (21.1528, -15.7821)
  line L174 (21.1528, -15.7821) -> (20.807, -15.7821)
  line L175 (20.807, -15.7821) -> (21.9951, -11.9363)
  line L176 (21.9951, -11.9363) -> (22.3458, -11.9363)
  line L177 (24.5614, -15.1202) -> (22.6817, -15.1202)
  line L178 (22.6817, -15.1202) -> (22.6817, -14.6879)
  spline S181 degree 2 poles (22.6817, -14.6879) (22.8843, -14.4977) (23.2449, -14.1445) (23.4178, -13.9543) knots 0 0 0 1 2 2 2
  spline S182 degree 2 poles (23.4178, -13.9543) (23.7661, -13.5715) (24.0205, -13.112) (24.0205, -12.8675) knots 0 0 0 1 2 2 2
  spline S183 degree 2 poles (24.0205, -12.8675) (24.0205, -12.7391) (23.9414, -12.5464) (23.8698, -12.4847) knots 0 0 0 1 2 2 2
  spline S184 degree 2 poles (23.8698, -12.4847) (23.7982, -12.4229) (23.6105, -12.3612) (23.4968, -12.3612) knots 0 0 0 1 2 2 2
  spline S185 degree 2 poles (23.4968, -12.3612) (23.3881, -12.3612) (23.1658, -12.4155) (23.0646, -12.4575) knots 0 0 0 1 2 2 2
  spline S186 degree 2 poles (23.0646, -12.4575) (22.9781, -12.4921) (22.8176, -12.5909) (22.7682, -12.6255) knots 0 0 0 1 2 2 2
  line L179 (22.7682, -12.6255) -> (22.7459, -12.6255)
  line L180 (22.7459, -12.6255) -> (22.7459, -12.1907)
  spline S187 degree 2 poles (22.7459, -12.1907) (22.8719, -12.129) (23.3239, -12.0079) (23.5265, -12.0079) knots 0 0 0 1 2 2 2
  spline S188 degree 2 poles (23.5265, -12.0079) (23.9538, -12.0079) (24.4354, -12.46) (24.4354, -12.8453) knots 0 0 0 1 2 2 2
  spline S189 degree 2 poles (24.4354, -12.8453) (24.4354, -13.0256) (24.3515, -13.3269) (24.2774, -13.4554) knots 0 0 0 1 2 2 2
  spline S190 degree 2 poles (24.2774, -13.4554) (24.2033, -13.5888) (23.9884, -13.8506) (23.8698, -13.9766) knots 0 0 0 1 2 2 2
  spline S191 degree 2 poles (23.8698, -13.9766) (23.6771, -14.1865) (23.2054, -14.636) (23.0646, -14.767) knots 0 0 0 1 2 2 2
  line L181 (23.0646, -14.767) -> (24.5614, -14.767)
  line L182 (24.5614, -14.767) -> (24.5614, -15.1202)
  spline S192 degree 2 poles (26.8659, -13.5962) (26.8659, -14.4162) (26.3892, -15.1844) (25.8927, -15.1844) knots 0 0 0 1 2 2 2
  spline S193 degree 2 poles (25.8927, -15.1844) (25.3889, -15.1844) (24.9171, -14.4014) (24.9171, -13.5986) knots 0 0 0 1 2 2 2
  spline S194 degree 2 poles (24.9171, -13.5986) (24.9171, -12.7737) (25.3938, -12.0104) (25.8927, -12.0104) knots 0 0 0 1 2 2 2
  spline S195 degree 2 poles (25.8927, -12.0104) (26.3942, -12.0104) (26.8659, -12.8008) (26.8659, -13.5962) knots 0 0 0 1 2 2 2
  spline S196 degree 2 poles (26.3423, -14.5249) (26.4016, -14.3742) (26.451, -13.9099) (26.451, -13.5962) knots 0 0 0 1 2 2 2
  spline S197 degree 2 poles (26.451, -13.5962) (26.451, -13.2825) (26.4016, -12.8206) (26.3398, -12.665) knots 0 0 0 1 2 2 2
  spline S198 degree 2 poles (26.3398, -12.665) (26.2781, -12.5094) (26.0632, -12.3488) (25.8927, -12.3488) knots 0 0 0 1 2 2 2
  spline S199 degree 2 poles (25.8927, -12.3488) (25.7223, -12.3488) (25.5025, -12.5094) (25.4383, -12.6699) knots 0 0 0 1 2 2 2
  spline S200 degree 2 poles (25.4383, -12.6699) (25.3765, -12.8255) (25.3321, -13.2998) (25.3321, -13.5986) knots 0 0 0 1 2 2 2
  spline S201 degree 2 poles (25.3321, -13.5986) (25.3321, -13.9197) (25.3716, -14.3495) (25.4358, -14.5175) knots 0 0 0 1 2 2 2
  spline S202 degree 2 poles (25.4358, -14.5175) (25.4951, -14.6756) (25.7149, -14.846) (25.8927, -14.846) knots 0 0 0 1 2 2 2
  spline S203 degree 2 poles (25.8927, -14.846) (26.0607, -14.846) (26.2805, -14.6854) (26.3423, -14.5249) knots 0 0 0 1 2 2 2
  line L183 (29.1359, -15.1202) -> (27.2562, -15.1202)
  line L184 (27.2562, -15.1202) -> (27.2562, -14.6879)
  spline S204 degree 2 poles (27.2562, -14.6879) (27.4587, -14.4977) (27.8194, -14.1445) (27.9923, -13.9543) knots 0 0 0 1 2 2 2
  spline S205 degree 2 poles (27.9923, -13.9543) (28.3405, -13.5715) (28.5949, -13.112) (28.5949, -12.8675) knots 0 0 0 1 2 2 2
  spline S206 degree 2 poles (28.5949, -12.8675) (28.5949, -12.7391) (28.5159, -12.5464) (28.4443, -12.4847) knots 0 0 0 1 2 2 2
  spline S207 degree 2 poles (28.4443, -12.4847) (28.3726, -12.4229) (28.1849, -12.3612) (28.0713, -12.3612) knots 0 0 0 1 2 2 2
  spline S208 degree 2 poles (28.0713, -12.3612) (27.9626, -12.3612) (27.7403, -12.4155) (27.639, -12.4575) knots 0 0 0 1 2 2 2
  spline S209 degree 2 poles (27.639, -12.4575) (27.5526, -12.4921) (27.392, -12.5909) (27.3426, -12.6255) knots 0 0 0 1 2 2 2
  line L185 (27.3426, -12.6255) -> (27.3204, -12.6255)
  line L186 (27.3204, -12.6255) -> (27.3204, -12.1907)
  spline S210 degree 2 poles (27.3204, -12.1907) (27.4464, -12.129) (27.8984, -12.0079) (28.1009, -12.0079) knots 0 0 0 1 2 2 2
  spline S211 degree 2 poles (28.1009, -12.0079) (28.5283, -12.0079) (29.0099, -12.46) (29.0099, -12.8453) knots 0 0 0 1 2 2 2
  spline S212 degree 2 poles (29.0099, -12.8453) (29.0099, -13.0256) (28.9259, -13.3269) (28.8518, -13.4554) knots 0 0 0 1 2 2 2
  spline S213 degree 2 poles (28.8518, -13.4554) (28.7777, -13.5888) (28.5628, -13.8506) (28.4443, -13.9766) knots 0 0 0 1 2 2 2
  spline S214 degree 2 poles (28.4443, -13.9766) (28.2516, -14.1865) (27.7798, -14.636) (27.639, -14.767) knots 0 0 0 1 2 2 2
  line L187 (27.639, -14.767) -> (29.1359, -14.767)
  line L188 (29.1359, -14.767) -> (29.1359, -15.1202)
  spline S215 degree 2 poles (31.47, -14.1322) (31.47, -14.3668) (31.3144, -14.7645) (31.1835, -14.8979) knots 0 0 0 1 2 2 2
  spline S216 degree 2 poles (31.1835, -14.8979) (31.0477, -15.0387) (30.7068, -15.1844) (30.5018, -15.1844) knots 0 0 0 1 2 2 2
  spline S217 degree 2 poles (30.5018, -15.1844) (30.2968, -15.1844) (29.9584, -15.0461) (29.83, -14.9077) knots 0 0 0 1 2 2 2
  spline S218 degree 2 poles (29.83, -14.9077) (29.6719, -14.7423) (29.494, -14.1865) (29.494, -13.7814) knots 0 0 0 1 2 2 2
  spline S219 degree 2 poles (29.494, -13.7814) (29.494, -13.3837) (29.6571, -12.744) (29.8275, -12.5069) knots 0 0 0 1 2 2 2
  spline S220 degree 2 poles (29.8275, -12.5069) (29.993, -12.2747) (30.5166, -12.0154) (30.8599, -12.0154) knots 0 0 0 1 2 2 2
  spline S221 degree 2 poles (30.8599, -12.0154) (30.9612, -12.0154) (31.1391, -12.0351) (31.2058, -12.0573) knots 0 0 0 1 2 2 2
  line L189 (31.2058, -12.0573) -> (31.2058, -12.4501)
  line L190 (31.2058, -12.4501) -> (31.1885, -12.4501)
  spline S222 degree 2 poles (31.1885, -12.4501) (31.1317, -12.4204) (30.9242, -12.3686) (30.8056, -12.3686) knots 0 0 0 1 2 2 2
  spline S223 degree 2 poles (30.8056, -12.3686) (30.4252, -12.3686) (29.9584, -12.8823) (29.9139, -13.3862) knots 0 0 0 1 2 2 2
  spline S224 degree 2 poles (29.9139, -13.3862) (30.0597, -13.2849) (30.3659, -13.1738) (30.5487, -13.1738) knots 0 0 0 1 2 2 2
  spline S225 degree 2 poles (30.5487, -13.1738) (30.7266, -13.1738) (30.9933, -13.2454) (31.1391, -13.3541) knots 0 0 0 1 2 2 2
  spline S226 degree 2 poles (31.1391, -13.3541) (31.307, -13.4801) (31.47, -13.8703) (31.47, -14.1322) knots 0 0 0 1 2 2 2
  spline S227 degree 2 poles (31.0551, -14.1495) (31.0551, -13.9617) (30.9563, -13.7073) (30.8476, -13.6184) knots 0 0 0 1 2 2 2
  spline S228 degree 2 poles (30.8476, -13.6184) (30.7661, -13.5542) (30.5635, -13.5122) (30.4573, -13.5122) knots 0 0 0 1 2 2 2
  spline S229 degree 2 poles (30.4573, -13.5122) (30.3141, -13.5122) (30.0448, -13.5986) (29.9139, -13.6801) knots 0 0 0 1 2 2 2
  spline S230 degree 2 poles (29.9139, -13.6801) (29.9115, -13.7246) (29.9065, -13.8086) (29.9065, -13.8728) knots 0 0 0 1 2 2 2
  spline S231 degree 2 poles (29.9065, -13.8728) (29.9065, -14.189) (30.03, -14.5768) (30.1239, -14.678) knots 0 0 0 1 2 2 2
  spline S232 degree 2 poles (30.1239, -14.678) (30.2103, -14.7744) (30.3981, -14.8509) (30.5043, -14.8509) knots 0 0 0 1 2 2 2
  spline S233 degree 2 poles (30.5043, -14.8509) (30.7513, -14.8509) (31.0551, -14.5002) (31.0551, -14.1495) knots 0 0 0 1 2 2 2
  point P0 (22, -11.35)
  point P1 (51.9257, -11.35)
  point P2 (22, -11.35)
  point P3 (22, -5.0636)
  dimension "d0" = 22.7
  dimension "d1" = 47
  constraints: 6 midpoint, 2 end point, 1 horizontal alignment, 1 vertical alignment, 2 other
extrude "Text" cut sketch "Sketch8" against normal blind 1 contours S68 S69 S70 L75 L76 L5 L79 S76 S77 S78 | L5 S78 S79 L79 L76 S71 S67 S68 | L5 S71 S72 S73 L77 L78 S74 S75 S67 | L176 L173 L5 | L5 L173 L174 L175 L176 | L8 L9 L10 L11 L12 L13 L14 L15 L16 L17 L18 L19 | L20 L21 L22 L23 L24 L25 L26 | S0 S1 S2 S3 L27 L28 S4 S5 S6 L29 L30 S7 S8 | L32 L33 S13 S14 S15 L34 L35 L36 L37 L38 S16 S17 L39 | S18 L40 L41 L42 L43 L44 L45 L46 L47 L48 L49 L50 S19 S20 S21 L51 L52 S22 | S23 S24 S25 S26 S27 S28 L53 L54 S29 S30 S31 S32 S33 S34 S35 S36 L55 L56 S37 S38 | S39 S40 S41 S42 S43 S44 L57 S45 S46 S47 L58 L59 S48 S49 S50 L60 L61 L62 | L64 S55 S56 S57 S58 L65 L66 L67 S59 S60 S61 L68 L69 L70 L71 L72 S62 S63 S64 S65 S66 L73 L74 | L80 S80 S81 L81 L82 L83 L84 L85 S82 S83 L86 | S84 S85 S86 S87 S88 S89 L87 S90 S91 S92 L88 L89 S93 S94 S95 L90 L91 L92 | L94 L95 L96 L97 L98 L99 L100 L101 | L105 L106 S100 S101 S102 S103 S104 S105 S106 L107 L108 L109 | S111 S112 S113 S114 S115 S116 L111 S117 S118 S119 L112 L113 S120 S121 S122 L114 L115 L116 | S127 S128 L118 L119 L120 L121 L122 S129 S130 | S135 L124 L125 L126 L127 L128 L129 L130 L131 L132 L133 L134 S136 S137 S138 L135 L136 S139 | S140 S141 S142 S143 L137 L138 S144 S145 S146 L139 L140 S147 S148 | L142 S153 S154 L143 L144 L145 L146 L147 S155 S156 L148 | S157 S158 S159 L149 L150 S160 S161 S162 S163 S164 S165 S166 L151 L152 L153 L154 L155 S167 S168 S169 | L156 L157 L158 L159 | L160 L161 S170 S171 S172 S173 S174 S175 L162 L163 S176 S177 S178 S179 S180 L164 L165 | L166 L167 L168 L169 L170 L171 L172 | L177 L178 S181 S182 S183 S184 S185 S186 L179 L180 S187 S188 S189 S190 S191 L181 L182 | S192 S193 S194 S195 | L183 L184 S204 S205 S206 S207 S208 S209 L185 L186 S210 S211 S212 S213 S214 L187 L188 | S215 S216 S217 S218 S219 S220 S221 L189 L190 S222 S223 S224 S225 S226
body "Solid1"
